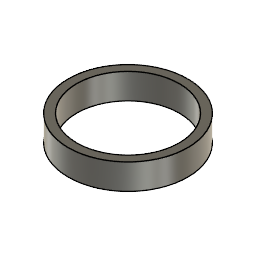
tire (Autodesk Fusion 360 design; units mm, degrees)
part number: 2026-05-16-10-16-58-379
Autodesk Fusion 360 part; units mm, degrees
sketch "Sketch1" plane through (0, 0, 0) normal (0, 0, 1) x (1, 0, 0)
  circle A0 centre (0, 0) radius 30.05
  circle A1 centre (0, 0) radius 35
  dimension "d1" = 60.1
  dimension "d2" = 70
  constraint coincident A0.centre A1.centre
  constraint concentric A0 A1
  measures "d1" diameter of A0
  measures "d2" diameter of A1
extrude "Extrude1" add sketch "Sketch1" along normal blind 15
